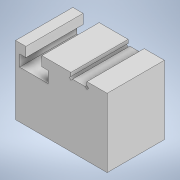
# Autodesk Inventor part: PiesaSuportCanale
Saved by Autodesk Inventor 2022 (Build 260153000, 153)
## iProperties
Created: 2022-03-05
Part Number: PiesaSuportCanale
Material: Generic
Document SubType Name: Modeling
Designer: Janina
Density: 1 g/cm^3
Appearance: Default
Author: Janina
Autodesk Inventor part; units mm, degrees
ref_plane "YZ Plane" through (0, 0, 0) normal (1, 0, 0) x (0, 1, 0)
ref_plane "XZ Plane" through (0, 0, 0) normal (0, 1, 0) x (-1, 0, 0)
ref_plane "XY Plane" through (0, 0, 0) normal (0, 0, 1) x (1, 0, 0)
sketch "Sketch1" plane through (0, 0, 0) normal (0, 0, 1) x (1, 0, 0)
  line L0 (-31.9403, 23.9801) -> (48.0597, 23.9801)
  line L1 (48.0597, 23.9801) -> (48.0597, -36.0199)
  line L2 (48.0597, -36.0199) -> (-31.9403, -36.0199)
  line L3 (-31.9403, -36.0199) -> (-31.9403, 23.9801)
  point P0 (0, 0)
  dimension "d0" = 80
  dimension "d1" = 60
  constraints: 8 end point, 2 parallel, 1 horizontal, 1 perpendicular
  measures "d0" distance of L0.start L0.end
  measures "d1" distance of L2.end L0.start
extrude "Extrusion1" add sketch "Sketch1" along normal blind 50
sketch "Sketch2" plane through (0, 0, 50) normal (0, 0, 1) x (1, 0, 0)
  line L0 (-22.9273, 24.546) -> (-8.9273, 24.546)
  line L1 (-8.9273, 24.546) -> (-8.9273, 15.546)
  line L2 (-8.9273, 15.546) -> (-3.4273, 15.546)
  line L3 (-3.4273, 15.546) -> (-3.4273, 5.546)
  line L4 (-3.4273, 5.546) -> (-28.4273, 5.546)
  line L5 (-28.4273, 5.546) -> (-28.4273, 15.546)
  line L6 (-28.4273, 15.546) -> (-22.9273, 15.546)
  line L7 (-22.9273, 15.546) -> (-22.9273, 24.546)
  point P0 (0, 0)
  point P1 (-15.9273, 24.546)
  dimension "d4" = 14
  dimension "d5" = 10
  dimension "d6" = 9
  dimension "d7" = 25
  dimension "d8" = 7
  dimension "d9" = 12.5
  constraints: 16 end point, 6 perpendicular, 2 point on line, 1 horizontal, 1 midpoint
  measures "d4" distance of L0.start L0.end
  measures "d5" distance of L4.end L5.end
  measures "d6" distance of L6.end L0.start
  measures "d7" distance of L3.end L4.end
  measures "d8" distance of L0.start point (-15.927, 24.546)
  measures "d9" distance from line of L5 point (-15.927, 24.546)
extrude "Extrusion2" cut sketch "Sketch2" against normal blind 50
sketch "Sketch3" plane through (0, 0, 50) normal (0, 0, 1) x (1, 0, 0)
  line L0 (23.4258, 24.5391) -> (30.4258, 24.5391)
  line L1 (30.4258, 24.5391) -> (30.4258, 20.9533)
  line L2 (30.4258, 20.9533) -> (31.84, 19.5391)
  line L3 (31.84, 19.5391) -> (30.4258, 18.1249)
  line L4 (30.4258, 18.1249) -> (29.0116, 19.5391)
  line L5 (29.0116, 19.5391) -> (23.4258, 19.5391)
  line L6 (23.4258, 24.5391) -> (23.4258, 19.5391) construction
  line L7 (23.4258, 24.5391) -> (16.4258, 24.5391)
  line L8 (16.4258, 24.5391) -> (16.4258, 20.9533)
  line L9 (16.4258, 20.9533) -> (15.0116, 19.5391)
  line L10 (15.0116, 19.5391) -> (16.4258, 18.1249)
  line L11 (16.4258, 18.1249) -> (17.84, 19.5391)
  line L12 (17.84, 19.5391) -> (23.4258, 19.5391)
  point P0 (0, 0)
  dimension "d12" = 7
  dimension "d13" = 5
  dimension "d14" = 2
  dimension "d15" = 135
  dimension "d16" = 2
  dimension "d18" = 2
  constraints: 26 end point, 5 symmetric about line, 3 coincident, 3 perpendicular, 1 horizontal, 1 parallel, 1 vertical
  measures "d12" distance of L0.start L0.end
  measures "d13" distance from line of L6.end L0
  measures "d14" distance of L2.end L3.end
  measures "d15" angle of L4 L5
  measures "d16" distance of L1.end L2.end
  measures "d18" distance of L3.end L4.end
extrude "Extrusion3" cut sketch "Sketch3" against normal blind 50
body "Solid1"
